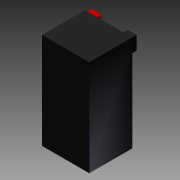
# Autodesk Inventor part: TB1272-Battery
Saved by Autodesk Inventor 2012 (Build 160160000, 160)
## iProperties
Created: 2013-07-14
Part Number: TB1272-Battery
Material: Lead
Document SubType Name: Modeling
Designer: joe_000
Density: 2.46917 g/cm^3
Mass: 1320 g
Surface Area: 437 cm^2
Volume: 534.592 cm^3
BatteryHeight: 60.000 mm
BatteryWidth: 66.000 mm
BatteryLength: 134.000 mm
Author: joe_000
Autodesk Inventor part; units mm, degrees
ref_plane "YZ Plane" through (0, 0, 0) normal (1, 0, 0) x (0, 1, 0)
ref_plane "XZ Plane" through (0, 0, 0) normal (0, 1, 0) x (-1, 0, 0)
ref_plane "XY Plane" through (0, 0, 0) normal (0, 0, 1) x (1, 0, 0)
sketch "Sketch1" plane through (0, 0, 0) normal (0, 0, 1) x (1, 0, 0)
  line L0 (0, 0) -> (66, 0)
  line L1 (66, 0) -> (66, 60)
  line L2 (66, 60) -> (0, 60)
  line L3 (0, 60) -> (0, 0)
  dimension "BatteryHeight" = 60
  dimension "BatteryWidth" = 66
  constraints: 8 end point, 2 parallel, 1 horizontal, 1 perpendicular
  measures "BatteryHeight" distance of L0.end L1.end
  measures "BatteryWidth" distance of L1.end L2.end
extrude "Extrusion1" add sketch "Sketch1" along normal blind 134
sketch "Sketch2" plane through (0, 60, 0) normal (0, 1, 0) x (1, 0, 0)
  line L0 (2, -132) -> (15, -132)
  line L1 (15, -132) -> (15, -113)
  line L2 (15, -113) -> (2, -113)
  line L3 (2, -113) -> (2, -132)
  line L4 (0, -134) -> (66, -134) projected
  line L5 (0, 0) -> (0, -134) projected
  dimension "d6" = 2
  dimension "d7" = 19
  dimension "d8" = 13
  dimension "d9" = 2
  constraints: 8 end point, 2 parallel, 1 horizontal, 1 perpendicular
  measures "d6" distance between parallel lines of L5 L3
  measures "d7" distance of L2.end L0.start
  measures "d8" distance of L1.end L2.end
  measures "d9" distance between parallel lines of L4 L0
extrude "Extrusion2" add sketch "Sketch2" along normal blind 8 separate body
sketch "Sketch3" plane through (0, 60, 0) normal (0, 1, 0) x (1, 0, 0)
  line L0 (0, -134) -> (66, -134) projected
  line L1 (66, 0) -> (66, -134) projected
  line L2 (64, -132) -> (51, -132)
  line L3 (51, -132) -> (51, -113)
  line L4 (51, -113) -> (64, -113)
  line L5 (64, -113) -> (64, -132)
  dimension "d10" = 19
  dimension "d11" = 13
  dimension "d12" = 2
  dimension "d13" = 2
  constraints: 8 end point, 2 parallel, 1 horizontal, 1 perpendicular
  measures "d10" distance of L4.end L2.start
  measures "d11" distance of L2.start L2.end
  measures "d12" distance between parallel lines of L0 L2
  measures "d13" distance between parallel lines of L1 L5
extrude "Extrusion3" add sketch "Sketch3" along normal blind 8 separate body
sketch "Sketch4" plane through (66, 0, 0) normal (1, 0, 0) x (0, 0, -1)
  line L0 (-134, 60) -> (-134, 0) projected
  line L1 (0, 0) -> (-134, 0) projected
  line L2 (0, 0) -> (0, 60) projected
  line L3 (0, 60) -> (-134, 60) projected
  line L4 (-67, 60) -> (-67, 0)
  constraints: 2 end point, 2 midpoint
sketch "Sketch5" plane through (0, 0, 0) normal (-1, 0, 0) x (0, 0, 1)
  line L0 (134, 0) -> (134, 60) projected
  line L1 (0, 60) -> (134, 60) projected
  line L2 (0, 60) -> (0, 0) projected
  line L3 (0, 0) -> (134, 0) projected
  line L4 (67, 60) -> (67, 0)
  constraints: 2 end point, 2 midpoint
body "Solid1"
body "Solid2"
body "Solid3"
